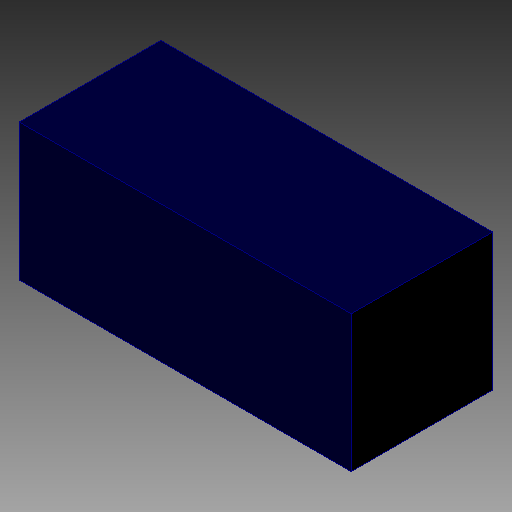
# Autodesk Inventor part: 0402
Saved by Autodesk Inventor 2018 (Build 220112000, 112)
## iProperties
Created: 2015-11-24
Part Number: 0402
Material: Generic
Document SubType Name: Modeling
Designer: PhillipD
Density: 1 g/cm^3
Appearance: 0402, 0402
Author: PhillipD
Autodesk Inventor part; units mm, degrees
ref_plane "YZ Plane" through (0, 0, 0) normal (1, 0, 0) x (0, 1, 0)
ref_plane "XZ Plane" through (0, 0, 0) normal (0, 1, 0) x (-1, 0, 0)
ref_plane "XY Plane" through (0, 0, 0) normal (0, 0, 1) x (1, 0, 0)
sketch "0402, 0402_1" plane through (0, 0, 0) normal (0, 0, 1) x (1, 0, 0)
  line L0 (-1.173, 0.483) -> (1.173, 0.483)
  line L1 (1.173, 0.483) -> (1.173, -0.483)
  line L2 (1.173, -0.483) -> (-1.173, -0.483)
  line L3 (-1.173, -0.483) -> (-1.173, 0.483)
  constraints: 8 end point
extrude "Extrusion1" add sketch "0402, 0402_1" along normal blind 1
body "Solid1"
